Laptop Holder Downer (Autodesk Fusion 360 design; units mm, degrees)
Autodesk Fusion 360 part; units mm, degrees
sketch "Sketch1" plane through (0, 0, 0) normal (0, 0, 1) x (1, 0, 0)
  circle A0 centre (0, 0) radius 2
  line L0 (0, 0) -> (-6, 0) construction
  arc A1 (-6, 0) -> (6, 0) centre (0, 0) ccw
  line L1 (6, 0) -> (6, 6)
  line L2 (6, 6) -> (-6, 6)
  line L3 (-6, 6) -> (-6, 0)
  line L4 (-6, 6) -> (-6, 10)
  line L5 (-6, 10) -> (6, 10)
  line L6 (6, 10) -> (6, 6)
  dimension "d1" = 4
  dimension "d2" = 4
  dimension "d3" = 4
  dimension "d4" = 6
  constraint coincident A0.centre L0.start
  constraint horizontal L0
  constraint tangent A1 L1
  constraint vertical L1
  constraint perpendicular L1 L2
  constraint tangent A1 L3
  constraint perpendicular L2 L4
  constraint perpendicular L1 L5
  constraint perpendicular L2 L6
  measures "d1" diameter of A0
  measures "d2" distance of A0 A1
  measures "d3" distance of L2 L5
  measures "d4" distance of A0.centre L2
extrude "Extrude1" add sketch "Sketch1" along normal blind 2 contours A1 L1 L2 L3 makes body 1
extrude "Extrude2" add sketch "Sketch1" along normal blind 19 contours L2 L4 L5 L6 bodies 1
sketch "Sketch2" plane through (6, 0, 0) normal (1, 0, 0) x (0, 1, 0)
  line L0 (0, 0) -> (10, 0)
  line L1 (10, 0) -> (10, 19)
  line L2 (10, 19) -> (6, 19)
  line L3 (6, 19) -> (6, 2)
  line L4 (6, 2) -> (0, 2)
  line L5 (0, 2) -> (0, 0)
sketch "Sketch3" plane through (6, 0, 0) normal (1, 0, 0) x (0, 1, 0)
  line L0 (0, 0) -> (10, 0)
  line L1 (10, 0) -> (10, 19)
  line L2 (10, 19) -> (6, 19)
  line L3 (6, 19) -> (6, 2)
  line L4 (6, 2) -> (0, 2)
  line L5 (0, 2) -> (0, 0)
  arc A0 (11, 18) -> (10, 19) centre (10, 18) ccw
  line L6 (11, 18) -> (10, 17)
  point P0 (10, 19)
  dimension "d11" = 45
  dimension "d12" = 2
  constraint coincident P0 L1.end
  constraint tangent L2 A0
  constraint coincident L1 L6.end
  constraint horizontal A0.start A0.centre
  measures "d11" angle of L1 L6
  measures "d12" distance of L6.end P0
extrude "Extrude3" add sketch "Sketch3" against normal blind 12 separate body contours L1 A0 L6 makes body 2
ref_plane "WorkPlane1" through (0, 8, 9.5) normal (0, 1, 0) x (-1, 0, 0)
mirror "Mirror1" about plane through (0, 8, 9.5) normal (0, 1, 0) of bodies 2 makes body 3
combine "Combine1" operation add target body 1 tool bodies 2 3
sketch "Sketch1 (2)" plane through (0, 0, 0) normal (1, 0, 0) x (0, 1, 0) in component "v2"
  line L0 (2, 2) -> (2, 0) construction
  line L1 (2, 0) -> (10, 0) construction
  line L2 (10, 0) -> (10, 17) construction
  line L3 (10, 17) -> (11, 18) construction
  arc A0 (11, 18) -> (10, 19) centre (10, 18) ccw construction
  line L4 (10, 19) -> (6, 19) construction
  arc A1 (6, 19) -> (5, 18) centre (6, 18) ccw construction
  line L5 (5, 18) -> (6, 17) construction
  line L6 (6, 17) -> (6, 2) construction
  line L7 (6, 2) -> (2, 2) construction
  line L8 (-6, 2) -> (-6, 0) construction
  line L9 (-6, 0) -> (-2, 0) construction
  line L10 (-2, 0) -> (-2, 2) construction
  line L11 (-2, 2) -> (-6, 2) construction
  line L12 (0, 0) -> (-20, 0) construction
  line L13 (-20, 0) -> (-20, 14)
  line L14 (-20, 14) -> (-25.7321, 14)
  line L15 (-20, 0) -> (-36, 0)
  line L16 (-36, 0) -> (-36, 2.5)
  line L17 (-24, 11) -> (-25.7321, 14)
  line L18 (-36, 2.5) -> (-24, 2.5)
  line L19 (-24, 2.5) -> (-24, 11)
  dimension "d17" = 20
  dimension "d18" = 14
  dimension "d20" = 2.5
  dimension "d23" = 4
  dimension "d24" = 150
  dimension "d25" = 3
  dimension "d26" = 16
  dimension "d27" = 4
  dimension "d28" = 4
  constraint coincident L12.start origin
  constraint perpendicular L10 L12
  constraint vertical L13
  constraint perpendicular L12 L13
  constraint perpendicular L13 L14
  constraint perpendicular L13 L15
  constraint perpendicular L15 L16
  constraint perpendicular L16 L18
  constraint vertical L19
  measures "d17" distance of L12.start L12.end
  measures "d18" distance of L12.end L13.end
  measures "d20" distance of L15.end L16.end
  measures "d23" distance of L13 L18.end
  measures "d24" angle of L17 L19
  measures "d25" distance of L14 L17.start
  measures "d26" distance of L12.end L15.end
  measures "d27" distance of L0.start L10.end
  measures "d28" distance of L0 L6
extrude "Extrude1'" add sketch "Sketch1 (2)" along normal mid plane 12 separate body makes body 4 in component "v2"
fillet "Fillet1" radius 2 1 edges at (0, -20, 14) on bodies 4 in component "v2"
sketch "Sketch2 (2)" plane through (0, 0, 2.5) normal (0, 0, 1) x (-1, 0, 0) in component "v2"
  line L0 (6, 36) -> (-6, 36)
  line L1 (-6, 36) -> (-6, 24)
  line L2 (-6, 24) -> (6, 24)
  line L3 (6, 24) -> (6, 36)
  line L4 (6, 24) -> (-6, 24)
  line L5 (0, 24) -> (0, 30) construction
  circle A0 centre (0, 30) radius 2
  line L6 (-2, 29.1716) -> (-2, 30.8284)
  line L7 (-2, 30) -> (0, 30)
  line L8 (-2, 29.1716) -> (-1.4142, 28.5858)
  line L9 (-2, 30.8284) -> (-1.4142, 31.4142)
  dimension "d33" = 6
  dimension "d34" = 4
  dimension "d39" = 90
  constraint midpoint L4 L5.start
  constraint perpendicular L4 L5
  constraint coincident L5.end A0.centre
  constraint vertical L6
  constraint midpoint L6 L7.start
  constraint horizontal L7
  constraint tangent A0 L6
  constraint coincident A0 L8.end
  constraint tangent A0 L8
  constraint coincident A0 L9.end
  constraint tangent A0 L9
  measures "d33" distance of L5.start L5.end
  measures "d34" diameter of A0
  measures "d39" angle of L8 L9
extrude "Extrude2'" cut sketch "Sketch2 (2)" against normal through all contours A0 | A0 L6 L9 | A0 L6 L8 bodies 4 in component "v2"
chamfer "Chamfer1" distance 0.4 angle 45 1 edges at (0, -25.7321, 14) on bodies 4 in component "v2"
fillet "Fillet2" radius 1 1 edges at (0, -24, 2.5) on bodies 4 in component "v2"
component "v2" placed x (1, 0, 0) y (0, 1, 0) z (0, 0, 1) at (0, 0, 0)
equation "d3 = d2"
named bodies: "v1", "v2"
